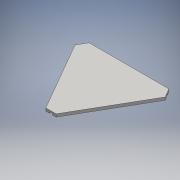
# Autodesk Inventor part: bottom plate
Saved by Autodesk Inventor 2016 SP1 (Build 200210100, 210)
## iProperties
Created: 2016-04-14
Part Number: bottom plate
Material: Generic
Document SubType Name: Modeling
Designer: ubik
Density: 1 g/cm^3
Appearance: Default
Author: ubik
Autodesk Inventor part; units mm, degrees
ref_plane "YZ Plane" through (0, 0, 0) normal (1, 0, 0) x (0, 1, 0)
ref_plane "XZ Plane" through (0, 0, 0) normal (0, 1, 0) x (-1, 0, 0)
ref_plane "XY Plane" through (0, 0, 0) normal (0, 0, 1) x (1, 0, 0)
sketch "Sketch1" plane through (0, 0, 0) normal (0, 0, 1) x (1, 0, 0)
  arc A0 (21.6973, 4.8506) -> (16.5011, 13.8506) centre (16.5011, 7.8506) ccw projected
  line L0 (21.6973, 4.8506) -> (13.3257, -9.6494) projected
  arc A1 (5.5315, -14.1494) -> (13.3257, -9.6494) centre (5.5315, -5.1494) ccw projected
  line L1 (5.5315, -14.1494) -> (-5.5315, -14.1494) projected
  arc A2 (-13.3257, -9.6494) -> (-5.5315, -14.1494) centre (-5.5315, -5.1494) ccw projected
  line L2 (-13.3257, -9.6494) -> (-21.6973, 4.8506) projected
  arc A3 (-16.5011, 13.8506) -> (-21.6973, 4.8506) centre (-16.5011, 7.8506) ccw projected
  line L3 (-16.5011, 13.8506) -> (16.5011, 13.8506) projected
  line L4 (-10, -40.5494) -> (-10, -20.5494) projected
  line L5 (-10, -20.5494) -> (10, -20.5494) projected
  line L6 (10, -20.5494) -> (10, -40.5494) projected
  line L7 (10, -40.5494) -> (-10, -40.5494) projected
  line L8 (15, -16.7494) -> (43, 31.7481) projected
  line L9 (43, 31.7481) -> (38.6699, 34.2481) projected
  line L10 (38.6699, 34.2481) -> (31.7143, 22.2006) projected
  arc A4 (23.4871, 17.4506) -> (31.7143, 22.2006) centre (23.4871, 26.9506) ccw projected
  line L11 (23.4871, 17.4506) -> (-23.4871, 17.4506) projected
  arc A5 (-31.7143, 22.2006) -> (-23.4871, 17.4506) centre (-23.4871, 26.9506) ccw projected
  line L12 (-31.7143, 22.2006) -> (-38.6699, 34.2481) projected
  line L13 (-38.6699, 34.2481) -> (-43, 31.7481) projected
  line L14 (-43, 31.7481) -> (-15, -16.7494) projected
  line L15 (-15, -16.7494) -> (-32.2735, -26.7222) projected
  arc A6 (-32.2735, -26.7222) -> (32.2735, -26.7222) centre (0, -5.7301) ccw projected
  line L16 (32.2735, -26.7222) -> (15, -16.7494) projected
  arc A7 (227.9453, 437.2441) -> (222.7491, 428.2441) centre (227.9453, 431.2441) ccw projected
  line L17 (227.9453, 437.2441) -> (244.6884, 437.2441) projected
  arc A8 (252.4827, 432.7441) -> (244.6884, 437.2441) centre (244.6884, 428.2441) ccw projected
  line L18 (252.4827, 432.7441) -> (258.0141, 423.1633) projected
  arc A9 (258.0141, 414.1633) -> (258.0141, 423.1633) centre (250.2199, 418.6633) ccw projected
  line L19 (258.0141, 414.1633) -> (249.6425, 399.6633) projected
  arc A10 (239.2502, 399.6633) -> (249.6425, 399.6633) centre (244.4464, 402.6633) ccw projected
  line L20 (239.2502, 399.6633) -> (222.7491, 428.2441) projected
  line L21 (283.1115, 432.4934) -> (265.791, 422.4934) projected
  line L22 (265.791, 422.4934) -> (255.791, 439.8139) projected
  line L23 (255.791, 439.8139) -> (273.1115, 449.8139) projected
  line L24 (273.1115, 449.8139) -> (283.1115, 432.4934) projected
  line L25 (250.0001, 442.2441) -> (194.0001, 442.2441) projected
  line L26 (194.0001, 442.2441) -> (194.0001, 437.2441) projected
  line L27 (194.0001, 437.2441) -> (207.9112, 437.2441) projected
  arc A11 (216.1385, 432.4941) -> (207.9112, 437.2441) centre (207.9112, 427.7441) ccw projected
  line L28 (216.1385, 432.4941) -> (239.6255, 391.8133) projected
  arc A12 (239.6255, 382.3133) -> (239.6255, 391.8133) centre (231.3983, 387.0633) ccw projected
  line L29 (239.6255, 382.3133) -> (232.6699, 370.2659) projected
  line L30 (232.6699, 370.2659) -> (237.0001, 367.7659) projected
  line L31 (237.0001, 367.7659) -> (265.0001, 416.2633) projected
  line L32 (265.0001, 416.2633) -> (282.2736, 406.2904) projected
  arc A13 (282.2736, 406.2904) -> (250.0001, 462.1898) centre (247.9571, 423.7441) ccw projected
  line L33 (250.0001, 462.1898) -> (250.0001, 442.2441) projected
  arc A14 (-249.6424, 399.6635) -> (-239.2501, 399.6635) centre (-244.4463, 402.6635) ccw projected
  line L34 (-249.6424, 399.6635) -> (-258.014, 414.1635) projected
  arc A15 (-258.014, 423.1635) -> (-258.014, 414.1635) centre (-250.2198, 418.6635) ccw projected
  line L35 (-258.014, 423.1635) -> (-252.4825, 432.7443) projected
  arc A16 (-244.6883, 437.2443) -> (-252.4825, 432.7443) centre (-244.6883, 428.2443) ccw projected
  line L36 (-244.6883, 437.2443) -> (-227.9452, 437.2443) projected
  arc A17 (-222.749, 428.2443) -> (-227.9452, 437.2443) centre (-227.9452, 431.2443) ccw projected
  line L37 (-222.749, 428.2443) -> (-239.2501, 399.6635) projected
  line L38 (-273.1113, 449.8142) -> (-255.7908, 439.8142) projected
  line L39 (-255.7908, 439.8142) -> (-265.7908, 422.4937) projected
  line L40 (-265.7908, 422.4937) -> (-283.1113, 432.4937) projected
  line L41 (-283.1113, 432.4937) -> (-273.1113, 449.8142) projected
  line L42 (-264.9999, 416.2635) -> (-237, 367.7661) projected
  line L43 (-237, 367.7661) -> (-232.6699, 370.2661) projected
  line L44 (-232.6699, 370.2661) -> (-239.6254, 382.3135) projected
  arc A18 (-239.6254, 391.8135) -> (-239.6254, 382.3135) centre (-231.3982, 387.0635) ccw projected
  line L45 (-239.6254, 391.8135) -> (-216.1383, 432.4943) projected
  arc A19 (-207.9111, 437.2443) -> (-216.1383, 432.4943) centre (-207.9111, 427.7443) ccw projected
  line L46 (-207.9111, 437.2443) -> (-193.9999, 437.2443) projected
  line L47 (-193.9999, 437.2443) -> (-193.9999, 442.2443) projected
  line L48 (-193.9999, 442.2443) -> (-249.9999, 442.2443) projected
  line L49 (-249.9999, 442.2443) -> (-249.9999, 462.19) projected
  arc A20 (-249.9999, 462.19) -> (-282.2735, 406.2907) centre (-247.957, 423.7443) ccw projected
  line L50 (-282.2735, 406.2907) -> (-264.9999, 416.2635) projected
  line L51 (-249.9999, 462.19) -> (250.0001, 462.1898)
  line L52 (282.2736, 406.2904) -> (32.2735, -26.7222)
  line L53 (-32.2735, -26.7222) -> (-282.2735, 406.2907)
  line L54 (-249.9999, 462.19) -> (-282.2735, 406.2907)
  line L55 (250.0001, 462.1898) -> (282.2736, 406.2904)
  line L56 (-32.2735, -26.7222) -> (32.2735, -26.7222)
  point P0 (0, 0)
  constraints: 12 end point, 1 parallel
extrude "Extrusion1" add sketch "Sketch1" along normal blind 18 contours L0 A1 L1 A2 L2 A3 L3 A0 | L56 L15 L14 L13 L12 A5 L11 A4 L10 L9 L8 L16 L6 L5 L4 | L4 L5 L6 L56 | L53 L50 L42 L43 L44 A18 L45 A19 L46 L47 L48 L49 L51 L33 L25 L26 L27 A11 L28 A12 L29 L30 L31 L32 L52 L16 L8 L9 L10 A4 L11 A5 L12 L13 L14 L15 | L54 L40 L39 L38 L49 L48 L47 L46 A19 L45 A18 L44 L43 L42 L50 | L32 L31 L30 L29 A12 L28 A11 L27 L26 L25 L33 L55 L23 L22 L21 | L54 L38 L39 L40 | L21 L22 L23 L55 | L17 A8 L18 A9 L19 A10 L20 A7 | L34 A15 L35 A16 L36 A17 L37 A14
sketch "Sketch2" plane through (0, 0, 0) normal (0, 0, -1) x (-1, 0, 0)
  line L0 (282.2735, 406.2907) -> (32.2735, -26.7222) projected
  line L1 (249.9999, 462.19) -> (282.2735, 406.2907) projected
  line L2 (-250.0001, 462.1898) -> (249.9999, 462.19) projected
  line L3 (-282.2736, 406.2904) -> (-250.0001, 462.1898) projected
  line L4 (-32.2735, -26.7222) -> (-282.2736, 406.2904) projected
  line L5 (32.2735, -26.7222) -> (-32.2735, -26.7222) projected
  line L6 (238.4529, 442.19) -> (259.1795, 406.2907)
  line L7 (270.7265, 426.2907) -> (9.1795, -26.7222)
  line L8 (20.7265, -6.7222) -> (-20.7265, -6.7222)
  line L9 (-9.1795, -26.7222) -> (-270.7266, 426.2904)
  line L10 (-259.1796, 406.2904) -> (-238.4531, 442.1898)
  line L11 (-261.5471, 442.1898) -> (261.5469, 442.19)
  point P0 (0, 0)
  dimension "d2" = 20
  constraints: 12 end point, 12 point on line
  measures "d2" distance between parallel lines of L2 L11
extrude "Extrusion2" cut sketch "Sketch2" against normal blind 8 contours L7 L6 L11 L1 | L5 L9 L8 L7 | L7 L8 L9 L10 L11 L6 | L10 L9 L3 L11
body "Solid1"
